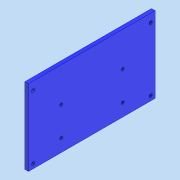
# Autodesk Inventor part: electronics_case_panel
Saved by Autodesk Inventor 2022 (Build 260153000, 153)
## iProperties
Created: 2022-01-17
Part Number: electronics_case_panel
Material: Generic
Document SubType Name: Modeling
Designer: nnico
Density: 1 g/cm^3
Appearance: Blue - Wall Paint - Glossy
Author: nnico
Autodesk Inventor part; units mm, degrees
ref_plane "YZ Plane" through (0, 0, 0) normal (1, 0, 0) x (0, 1, 0)
ref_plane "XZ Plane" through (0, 0, 0) normal (0, 1, 0) x (-1, 0, 0)
ref_plane "XY Plane" through (0, 0, 0) normal (0, 0, 1) x (1, 0, 0)
sketch "Sketch1" plane through (0, 0, 0) normal (1, 0, 0) x (0, 1, 0)
  line L0 (42, 70) -> (-42, 70)
  line L1 (-42, 70) -> (-42, -70)
  line L2 (-42, -70) -> (42, -70)
  line L3 (42, -70) -> (42, 70)
  line L4 (0, 70) -> (0, -70) construction
  line L5 (-42, 0) -> (42, 0) construction
  circle A0 centre (-37, 65) radius 1.75
  circle A1 centre (-37, -65) radius 1.75
  circle A2 centre (33, 65) radius 1.75
  circle A3 centre (-37, -65) radius 1.75
  circle A4 centre (33, -65) radius 1.75
  point P0 (0, 0)
  point P1 (0, 0)
  dimension "d0" = 84
  dimension "d1" = 140
  dimension "d2" = 3.5
  dimension "d3" = 5
  dimension "d4" = 5
  dimension "d5" = 3.5
  dimension "d6" = 9
  dimension "d7" = 5
  constraints: 12 end point, 5 centre point, 5 midpoint, 3 symmetric about line, 2 parallel, 1 coincident, 1 horizontal, 1 perpendicular, 3 other
  measures "d0" distance of L0.start L0.end
  measures "d1" distance of L2.end L0.start
  measures "d2" diameter of A0
  measures "d3" distance from line of L1 A0.centre
  measures "d4" distance from line of L0 A0.centre
  measures "d5" diameter of A2
  measures "d6" distance from line of L3 A2.centre
  measures "d7" distance from line of L0 A2.centre
extrude "Extrusion1" add sketch "Sketch1" along normal blind 4
sketch "Sketch2" plane through (4, 0, 0) normal (1, 0, 0) x (0, 0, -1)
  line L0 (-34, 4) -> (34, 4) construction
  line L1 (34, 4) -> (34, -28) construction
  line L2 (34, -28) -> (-34, -28) construction
  line L3 (-34, -28) -> (-34, 4) construction
  line L4 (-70, 42) -> (-70, -42) construction
  line L5 (70, 42) -> (-70, 42) construction
  line L6 (0, 42) -> (0, -42) construction
  line L7 (-70, -42) -> (70, -42) construction
  circle A0 centre (-34, -28) radius 1.5
  circle A1 centre (-34, 4) radius 1.5
  circle A2 centre (34, 4) radius 1.5
  circle A3 centre (34, -28) radius 1.5
  point P0 (0, 0)
  dimension "d10" = 36
  dimension "d11" = 32
  dimension "d12" = 14
  dimension "d13" = 3
  dimension "d14" = 3
  dimension "d15" = 3
  dimension "d16" = 3
  constraints: 10 end point, 4 centre point, 4 coincident, 2 parallel, 1 horizontal, 1 midpoint, 1 perpendicular, 1 vertical, 1 other
  measures "d10" distance from line of L4 L0.start
  measures "d11" distance of L2.end L0.start
  measures "d12" distance from line of L7 L2.end
  measures "d13" diameter of A0
  measures "d14" diameter of A1
  measures "d15" diameter of A2
  measures "d16" diameter of A3
extrude "Extrusion2" cut sketch "Sketch2" against normal blind 4
body "Solid1"
